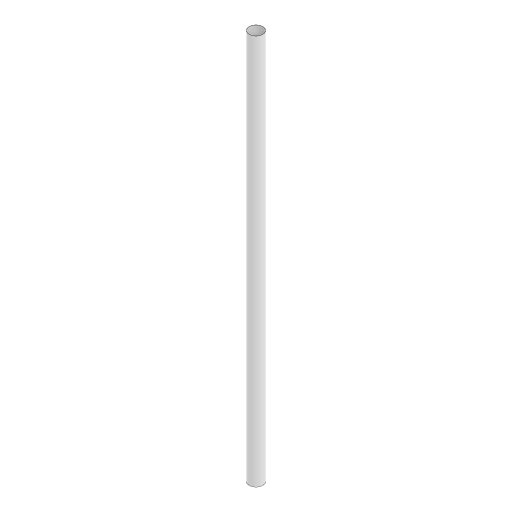
# Autodesk Inventor part: dummy_mckibben_pam_sleeve_4.2mm
Saved by Autodesk Inventor 2024.3 (Build 283343000, 343)
## iProperties
Created: 2024-09-12
Part Number: dummy_mckibben_pam_sleeve_4.2mm
Material: Generic
Document SubType Name: Modeling
Designer: gihyeok2
Density: 1 g/cm^3
Appearance: Default
Author: gihyeok2
Autodesk Inventor part; units mm, degrees
ref_plane "YZ Plane" through (0, 0, 0) normal (1, 0, 0) x (0, 1, 0)
ref_plane "XZ Plane" through (0, 0, 0) normal (0, 1, 0) x (-1, 0, 0)
ref_plane "XY Plane" through (0, 0, 0) normal (0, 0, 1) x (1, 0, 0)
sketch "Sketch1" plane through (0, 0, 0) normal (0, 1, 0) x (-1, 0, 0)
  circle A0 centre (0, 0) radius 2.05
  circle A1 centre (0, 0) radius 2.1
  dimension "d0" = 4.1
  dimension "d1" = 4.2
  constraints: 2 centre point, 2 coincident
  measures "d0" diameter of A0
  measures "d1" diameter of A1
extrude "Extrusion1" add sketch "Sketch1" along normal blind 120
body "Solid1"
